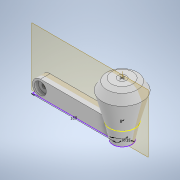
# Autodesk Inventor part: handle
Saved by Autodesk Inventor 2021 (Build 250183000, 183)
## iProperties
Created: 2021-03-11
Part Number: handle
Material: Generic
Document SubType Name: Modeling
Designer: ben
Density: 1 g/cm^3
Appearance: Default
Author: ben
Autodesk Inventor part; units mm, degrees
ref_plane "YZ Plane" through (0, 0, 0) normal (1, 0, 0) x (0, 1, 0)
ref_plane "XZ Plane" through (0, 0, 0) normal (0, 1, 0) x (-1, 0, 0)
ref_plane "XY Plane" through (0, 0, 0) normal (0, 0, 1) x (1, 0, 0)
sketch "Sketch1" plane through (0, 0, 0) normal (0, 0, 1) x (1, 0, 0)
  line L0 (25, -9) -> (-135, -9)
  line L1 (-135, -9) -> (-135, 9)
  line L2 (-135, 9) -> (25, 9)
  line L3 (25, 9) -> (25, -9)
  circle A0 centre (-135, 0) radius 17.5
  point P0 (0, 0)
  dimension "d0" = 160
  dimension "d1" = 18
  dimension "d5" = 35
  constraints: 8 end point, 2 parallel, 1 centre point, 1 horizontal, 1 midpoint, 1 perpendicular
  measures "d0" distance of L1.end L2.end
  measures "d1" distance of L0.end L1.end
  measures "d5" diameter of A0
extrude "Extrusion1" add sketch "Sketch1" along normal blind 30 contours L0 A0 L2 L3 | L0 L1 L2 A0 picked at (-129.1667, 0)
fillet "Fillet1" radius 15 2 edges at (25, 0, 30) (25, 0, 0)
sketch "Sketch9" plane through (10, 9, 15) normal (0, 1, 0) x (1, 0, 0)
  circle A0 centre (0, 0) radius 11.2
  point P0 (-10, 15)
  dimension "d21" = 22.4
  constraints: 1 centre point
  measures "d21" diameter of A0
extrude "Extrusion8" cut sketch "Sketch9" against normal through all
ref_plane "Work Plane4" through (10, 0, 15) normal (0, 1, 0) x (1, 0, 0)
sketch "Sketch19" plane through (10, 0, 15) normal (0, 1, 0) x (1, 0, 0)
  circle A0 centre (0, 0) radius 11.2 projected
  circle A1 centre (0, 0) radius 4
  point P0 (-10, 15)
  dimension "d59" = 8
  constraints: 1 centre point, 1 coincident
  measures "d59" diameter of A1
extrude "Extrusion19" add sketch "Sketch19" along normal mid plane 4
sketch "Sketch23" plane through (10, 0, 15) normal (0, 1, 0) x (1, 0, 0)
  line L0 (-121.0999, -15) -> (-107.7025, -65)
  line L1 (-107.7025, -65) -> (-116.3627, -80)
  line L2 (-116.3627, -80) -> (-125.023, -85)
  line L3 (-125.023, -85) -> (-141, -85)
  line L4 (-121.0999, -15) -> (-133.8, -15)
  line L5 (-145, -15) -> (0, -15) projected
  line L6 (-133.8, -15) -> (-133.8, -22.4)
  line L7 (-133.8, -22.4) -> (-141, -22.4)
  line L8 (-141, -22.4) -> (-141, -85)
  line L9 (-145, -105) -> (-145, 35) projected
  line L10 (-141, -83) -> (-137, -83)
  line L11 (-137, -83) -> (-137, -85)
  line L12 (-139, -83) -> (-139, -75)
  line L13 (-139, -83) -> (-131, -83) construction
  line L14 (-139, -75) -> (-141, -75)
  point P0 (-10, 15)
  dimension "d64" = 75
  dimension "d65" = 50
  dimension "d66" = 15
  dimension "d67" = 135
  dimension "d68" = 5
  dimension "d69" = 150
  dimension "d70" = 7.4
  dimension "d72" = 7.2
  dimension "d74" = 4
  dimension "d75" = 2
  dimension "d76" = 8
  dimension "d82" = 11.2
  dimension "d83" = 23.9001
  dimension "d98" = 0
  constraints: 26 end point, 5 horizontal, 4 perpendicular, 3 point on line, 2 vertical, 1 midpoint
  measures "d64" angle of L5 L0
  measures "d65" vertical distance of L0.start L0.end
  measures "d66" vertical distance of L1.end L0.end
  measures "d67" angle of L0 L1
  measures "d68" vertical distance of L2.end L1.end
  measures "d69" angle of L1 L2
  measures "d70" distance of L4.end L6.end
  measures "d72" distance of L6.end L7.end
  measures "d74" distance of L10.start L10.end
  measures "d75" distance of L10.end L11.end
  measures "d76" distance of L12.start L12.end
  measures "d82" distance between parallel lines of L9 L6
  measures "d83" distance of L5.start L0.start
  measures "d98" distance between parallel lines of L4 L5
sketch "Sketch26" plane through (10, 0, 15) normal (0, 1, 0) x (1, 0, 0)
  line L0 (-162.5, 15) -> (-127.5, 15) projected
  line L1 (-127.5, 15) -> (-121.0999, -15)
  line L2 (-145, 15) -> (-145, -15) projected
  line L3 (-121.0999, -15) -> (-145, -15)
  line L4 (-145, -15) -> (-145, 15)
  line L5 (-145, 15) -> (-127.5, 15)
  line L6 (-145, -105) -> (-145, 35) projected
  point P0 (-10, 15)
  constraints: 8 end point, 2 collinear, 1 horizontal
revolve "Revolution2" add sketch "Sketch26" angle 360 about axis through (-135, 0, 30) along (0, 0, -1)
sketch "Sketch27" plane through (-135, 0, 30) normal (0, 0, 1) x (0, -1, 0)
  circle A0 centre (0, 0) radius 4
  circle A1 centre (0, 0) radius 23.9001 projected
  dimension "d79" = 8
  constraints: 1 centre point
  measures "d79" diameter of A0
extrude "Extrusion21" add sketch "Sketch27" along normal blind 60 contours A0
revolve "Revolution3" add sketch "Sketch23" angle 360 about axis through (-135, 0, 30) along (0, 0, -1) separate body contours L0 L1 L2 L3 L11 L10 L12 L14 L8 L7 L6 L4
thread "Thread1" size "M12x1.75" class "6H" standard "ANSI Metric M Profile" full length
sketch "Sketch28" plane through (10, 0, 15) normal (0, 1, 0) x (1, 0, 0)
  line L0 (-153, -85) -> (-137, -85) projected
  line L1 (-153, -83) -> (-137, -83) projected
  line L2 (-151, -83) -> (-139, -83) projected
  line L3 (-151, -75) -> (-139, -75) projected
  line L4 (-137, -85) -> (-137, -83) projected
  line L5 (-153, -85) -> (-153, -83) projected
  line L6 (-151, -83) -> (-151, -75) projected
  line L7 (-139, -83) -> (-139, -75) projected
  line L8 (-145, -105) -> (-145, 35) projected
  point P0 (-10, 15)
  point P1 (-145, -75)
  point P2 (-145, -85)
revolve "Revolution4" add sketch "Sketch28" angle 360 about axis through (-135, 0, 30) along (0, 0, -1) separate body contours L8 L1 L4 L0 | L8 L3 L7 L1
thread "Thread2" size "M12x1.75" class "6g" standard "ANSI Metric M Profile" full length
sketch "Sketch29" plane through (-135, 0, 100) normal (0, 0, 1) x (1, 0, 0)
  line L0 (4, -0.5) -> (-4, -0.5)
  line L1 (-4, -0.5) -> (-4, 0.5)
  line L2 (-4, 0.5) -> (4, 0.5)
  line L3 (4, 0.5) -> (4, -0.5)
  line L4 (4, -0.5) -> (-4, 0.5) construction
  line L5 (-4, -0.5) -> (4, 0.5) construction
  line L6 (0.5, 4) -> (-0.5, 4)
  line L7 (-0.5, 4) -> (-0.5, -4)
  line L8 (-0.5, -4) -> (0.5, -4)
  line L9 (0.5, -4) -> (0.5, 4)
  line L10 (0.5, 4) -> (-0.5, -4) construction
  line L11 (-0.5, 4) -> (0.5, -4) construction
  point P0 (135, 0)
  point P1 (0, 0)
  point P2 (0, 0)
  point P3 (0, 0)
  point P4 (0, 0)
  point P5 (0, 0)
  point P6 (0, 0)
  point P7 (0.5, 0.5)
  point P8 (-0.5, 0.5)
  point P9 (-0.5, -0.5)
  point P10 (0.5, -0.5)
  dimension "d92" = 8
  dimension "d93" = 1
  dimension "d94" = 1
  dimension "d95" = 8
  constraints: 24 end point, 7 midpoint, 4 parallel, 2 coincident, 2 horizontal, 2 perpendicular
  measures "d92" distance of L1.end L2.end
  measures "d93" distance of L0.end L1.end
  measures "d94" distance of L8.end L7.end
  measures "d95" distance of L7.end L6.end
extrude "Extrusion22" cut sketch "Sketch29" against normal blind 2 bodies 3
